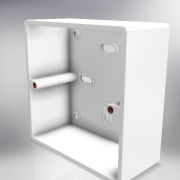
# Autodesk Inventor part: EJB1
Saved by Autodesk Inventor 2020 (Build 240168000, 168)
## iProperties
Created: 2021-02-04
Part Number: EJB1
Material: ABS Plastic
Document SubType Name: Modeling
Designer: Sikesh Bhivah
Mass: 50.6029 g
Surface Area: 410.777 cm^2
Volume: 47.7386 cm^3
Density: 1.06 g/cm^3
Appearance: White
Categories: <MemberInstance><Categories><Category DisplayName="" Mnemonic="IDF" InternalName="690189fb-5335-48bc-ba8f-fa4ddabb13bb"><Category DisplayName="" Mnemonic="COMPONENTS" InternalName="eab5d76b-1861-4102-82a0-277eae840d4a"><Category DisplayName="" Mnemonic="ELECTRICAL" InternalName="e935d458-c05c-4f25-8523-65af19dfc39b"/></Category></Category></Categories><FamilyTemplate><FamilyTemplateParameters></FamilyTemplateParameters></FamilyTemplate><CategoryParameterMap><ParamToTemplateMap></ParamToTemplateMap></CategoryParameterMap></MemberInstance>
Author: Sikesh Bhivah
Autodesk Inventor part; units mm, degrees
ref_plane "YZ Plane" through (0, 0, 0) normal (1, 0, 0) x (0, 1, 0)
ref_plane "XZ Plane" through (0, 0, 0) normal (0, 1, 0) x (-1, 0, 0)
ref_plane "XY Plane" through (0, 0, 0) normal (0, 0, 1) x (1, 0, 0)
sketch "Sketch1" plane through (0, 0, 0) normal (0, 0, 1) x (1, 0, 0)
  line L0 (-40, -43) -> (40, -43)
  line L1 (43, -40) -> (43, 40)
  line L2 (40, 43) -> (-40, 43)
  line L3 (-43, 40) -> (-43, -40)
  line L4 (-43, -43) -> (43, 43) construction
  line L5 (43, -43) -> (-43, 43) construction
  arc A0 (-40, 43) -> (-43, 40) centre (-40, 40) ccw
  arc A1 (43, 40) -> (40, 43) centre (40, 40) ccw
  arc A2 (40, -43) -> (43, -40) centre (40, -40) ccw
  arc A3 (-43, -40) -> (-40, -43) centre (-40, -40) ccw
  point P0 (0, 0)
  dimension "d0" = 86
  dimension "d1" = 3
  dimension "d16" = 86
  constraints: 12 end point, 8 point on circle, 8 point on line, 8 tangent, 4 centre point, 3 equal radius, 2 midpoint, 2 parallel, 1 horizontal, 1 perpendicular
  measures "d0" distance of L4.end L5.end
  measures "d1" radius of A0
  measures "d16" distance between parallel lines of L0 L2
extrude "Extrusion1" add sketch "Sketch1" along normal blind 3
sketch "Sketch2" plane through (0, 0, 3) normal (0, 0, 1) x (1, 0, 0)
  arc A0 (-40, 43) -> (-43, 40) centre (-40, 40) ccw projected
  line L0 (-43, 40) -> (-43, -40) projected
  arc A1 (-43, -40) -> (-40, -43) centre (-40, -40) ccw projected
  line L1 (-40, -43) -> (40, -43) projected
  arc A2 (40, -43) -> (43, -40) centre (40, -40) ccw projected
  line L2 (43, -40) -> (43, 40) projected
  arc A3 (43, 40) -> (40, 43) centre (40, 40) ccw projected
  line L3 (40, 43) -> (-40, 43) projected
  line L4 (-40, -40) -> (-40, 40)
  line L5 (-40, 40) -> (40, 40)
  line L6 (40, 40) -> (40, -40)
  line L7 (40, -40) -> (-40, -40)
  arc A4 (-34, -3) -> (-34, 3) centre (-34, 0) ccw
  arc A5 (34, 3) -> (34, -3) centre (34, 0) ccw
  line L8 (-34, 3) -> (-40, 3)
  line L9 (-34, -3) -> (-40, -3)
  line L10 (34, 3) -> (40, 3)
  line L11 (34, -3) -> (40, -3)
  arc A6 (-34, 3) -> (-34, -3) centre (-34, 0) ccw construction
  arc A7 (34, -3) -> (34, 3) centre (34, 0) ccw construction
  point P0 (0, 0)
  point P1 (40, 0)
  dimension "d4" = 3
  dimension "d5" = 6
  dimension "d6" = 6
  constraints: 16 end point, 10 point on circle, 10 point on line, 4 centre point, 2 equal length, 2 horizontal alignment, 2 perpendicular, 1 equal radius, 1 midpoint, 1 tangent, 3 other
  measures "d4" distance between parallel lines of L0 L4
  measures "d5" diameter of A5
  measures "d6" distance of point (40, 0) A5.centre
extrude "Extrusion2" add sketch "Sketch2" along normal blind 35 contours L3 A3 L2 A2 L1 A1 L0 A0 | L4 L8 A4 L9 | L11 A5 L10 L6
sketch "Sketch3" plane through (0, 0, 38) normal (0, 0, 1) x (1, 0, 0)
  arc A0 (-34, -3) -> (-34, 3) centre (-34, 0) ccw projected
  arc A1 (34, 3) -> (34, -3) centre (34, 0) ccw projected
  arc A2 (-34, -3) -> (-34, 3) centre (-34, 0) ccw projected
  point P0 (0, 0)
  constraints: 2 coincident
hole "Hole1" at (-34, 0, 38) at (34, 0, 38) direction (0, 0, -1) diameter 2.459 depth 18 tip angle 118 countersink diameter 4 countersink angle 90 thread size "M3x0.5" class "6H" standard "ISO Metric profile"
chamfer "Chamfer1" distance 0.3 angle 45 28 edges at (0, 43, 38) (-42.1213, 42.1213, 38) (-43, 0, 38) (-42.1213, -42.1213, 38) (0, -43, 38) (42.1213, -42.1213, 38) (43, 0, 38) (42.1213, 42.1213, 38) (0, 40, 38) (-40, 21.5, 38) (-31, 0, 38) (-37, 3, 38) (-37, -3, 38) (-40, -21.5, 38) (0, -40, 38) (40, -21.5, 38) (40, 21.5, 38) (37, 3, 38) (31, 0, 38) (37, -3, 38) (43, 0, 0) (42.1213, 42.1213, 0) (0, 43, 0) (-42.1213, 42.1213, 0) (-43, 0, 0) (-42.1213, -42.1213, 0) (0, -43, 0) (42.1213, -42.1213, 0)
sketch "Sketch4" plane through (0, 0, 0) normal (0, 0, -1) x (-1, 0, 0)
  line L0 (-8, 21) -> (-4, 21) construction
  line L1 (8, 21) -> (8, 29) construction
  line L2 (8, 29) -> (4, 29) construction
  line L3 (-8, 29) -> (-8, 21) construction
  line L4 (-8, 21) -> (8, 29) construction
  line L5 (8, 21) -> (-8, 29) construction
  line L6 (0, 0) -> (0, 25) construction
  arc A0 (-4, 29) -> (-4, 21) centre (-4, 25) ccw
  line L7 (-4, 21) -> (4, 21)
  line L8 (-4, 29) -> (-8, 29) construction
  arc A1 (-4, 21) -> (-4, 29) centre (-4, 25) ccw construction
  arc A2 (4, 21) -> (4, 29) centre (4, 25) ccw
  line L9 (4, 29) -> (-4, 29)
  line L10 (4, 21) -> (8, 21) construction
  line L11 (-42.7, -40) -> (-42.7, 40) projected
  arc A3 (-42.7, -40) -> (-40, -42.7) centre (-40, -40) ccw projected
  line L12 (40, -42.7) -> (-40, -42.7) projected
  arc A4 (40, -42.7) -> (42.7, -40) centre (40, -40) ccw projected
  line L13 (42.7, 40) -> (42.7, -40) projected
  arc A5 (42.7, 40) -> (40, 42.7) centre (40, 40) ccw projected
  line L14 (-40, 42.7) -> (40, 42.7) projected
  arc A6 (-40, 42.7) -> (-42.7, 40) centre (-40, 40) ccw projected
  line L15 (-39.7, 39.7) -> (-39.7, -39.7)
  line L16 (-39.7, -39.7) -> (39.7, -39.7)
  line L17 (39.7, -39.7) -> (39.7, 39.7)
  line L18 (39.7, 39.7) -> (-39.7, 39.7)
  line L19 (0, -39.7) -> (0, -34) construction
  line L20 (-4, -29) -> (4, -29) construction
  line L21 (4, -29) -> (4, -25) construction
  line L22 (4, -13) -> (-4, -13) construction
  line L23 (-4, -13) -> (-4, -17) construction
  line L24 (-4, -29) -> (4, -13) construction
  line L25 (4, -29) -> (-4, -13) construction
  arc A7 (-4, -17) -> (4, -17) centre (0, -17) ccw construction
  line L26 (4, -17) -> (4, -13) construction
  arc A8 (4, -17) -> (-4, -17) centre (0, -17) ccw
  arc A9 (-4, -25) -> (4, -25) centre (0, -25) ccw
  line L27 (-4, -17) -> (-4, -25)
  line L28 (-4, -25) -> (-4, -29) construction
  line L29 (4, -25) -> (4, -17)
  line L30 (0, 0) -> (0, -13) construction
  circle A10 centre (-31.7, 31.7) radius 4
  circle A11 centre (31.7, 31.7) radius 4
  line L31 (-21, -8) -> (-21, -4) construction
  line L32 (-21, 8) -> (-29, 8) construction
  line L33 (-29, 8) -> (-29, 4) construction
  line L34 (-21, -4) -> (-21, 4)
  line L35 (-29, 4) -> (-29, -4)
  line L36 (-29, -8) -> (-21, -8) construction
  line L37 (-29, -4) -> (-29, -8) construction
  line L38 (-21, 8) -> (-29, -8) construction
  arc A12 (-29, -4) -> (-21, -4) centre (-25, -4) ccw
  arc A13 (-21, -4) -> (-29, -4) centre (-25, -4) ccw construction
  line L39 (-21, -8) -> (-29, 8) construction
  line L40 (-21, 4) -> (-21, 8) construction
  arc A14 (-21, 4) -> (-29, 4) centre (-25, 4) ccw
  line L41 (0, 0) -> (-25, 0) construction
  line L42 (0, 0) -> (13, 0) construction
  line L43 (13, -4) -> (17, -4) construction
  arc A15 (17, 4) -> (17, -4) centre (17, 0) ccw
  line L44 (13, 4) -> (13, -4) construction
  arc A16 (17, -4) -> (17, 4) centre (17, 0) ccw construction
  line L45 (17, 4) -> (13, 4) construction
  line L46 (17, -4) -> (25, -4)
  line L47 (25, 4) -> (17, 4)
  line L48 (29, -4) -> (13, 4) construction
  line L49 (29, 4) -> (13, -4) construction
  line L50 (25, -4) -> (29, -4) construction
  line L51 (29, -4) -> (29, 4) construction
  arc A17 (25, -4) -> (25, 4) centre (25, 0) ccw
  line L52 (29, 4) -> (25, 4) construction
  circle A18 centre (-31.7, -31.7) radius 4
  circle A19 centre (31.7, -31.7) radius 4
  point P0 (0, -21)
  point P1 (0, -21)
  point P2 (0, 21)
  point P3 (-21, 0)
  point P4 (21, 0)
  point P5 (21, 0)
  dimension "d20" = 8
  dimension "d24" = 4
  dimension "d25" = 25
  dimension "d30" = 13
  dimension "d36" = 3
  dimension "d37" = 8
  dimension "d44" = 90
  dimension "d56" = 8
  dimension "d57" = 8
  constraints: 98 end point, 28 tangent, 27 point on circle, 20 parallel, 16 centre point, 12 midpoint, 6 perpendicular, 6 symmetric about line, 4 horizontal, 3 equal length, 2 equal radius, 1 coincident, 1 vertical, 1 vertical alignment, 63 other
  measures "d20" distance of A2.centre A0.centre
  measures "d24" radius of A0
  measures "d25" distance of L6.start point (0, 25)
  measures "d30" distance of L6.start L30.end
  measures "d36" distance between parallel lines of L11 L15
  measures "d37" diameter of A10
  measures "d56" distance from line of L18 A10.centre
  measures "d57" distance from line of L15 A10.centre
extrude "Extrusion3" cut sketch "Sketch4" against normal blind 1 contours L18 L17 L16 L15 | A18 | A19
sketch "Sketch5" plane through (0, 0, 3) normal (0, 0, 1) x (1, 0, 0)
  line L0 (4, 21) -> (-4, 21) projected
  arc A0 (-4, 29) -> (-4, 21) centre (-4, 25) ccw projected
  line L1 (-4, 29) -> (4, 29) projected
  arc A1 (4, 21) -> (4, 29) centre (4, 25) ccw projected
  circle A2 centre (-31.7, 31.7) radius 4 projected
  arc A3 (4, -17) -> (-4, -17) centre (0, -17) ccw projected
  line L2 (4, -17) -> (4, -25) projected
  arc A4 (-4, -25) -> (4, -25) centre (0, -25) ccw projected
  line L3 (-4, -25) -> (-4, -17) projected
  circle A5 centre (31.7, 31.7) radius 4 projected
  circle A6 centre (31.9662, -31.9095) radius 4 projected
  circle A7 centre (-31.9662, -31.9095) radius 4 projected
  line L4 (-40, 40) -> (-40, 3) projected
  line L5 (-40, 3) -> (-34, 3) projected
  arc A8 (-34, -3) -> (-34, 3) centre (-34, 0) ccw projected
  line L6 (-34, -3) -> (-40, -3) projected
  line L7 (-40, -3) -> (-40, -40) projected
  line L8 (-40, -40) -> (40, -40) projected
  line L9 (40, -40) -> (40, -3) projected
  line L10 (40, -3) -> (34, -3) projected
  arc A9 (34, 3) -> (34, -3) centre (34, 0) ccw projected
  line L11 (34, 3) -> (40, 3) projected
  line L12 (40, 3) -> (40, 40) projected
  line L13 (40, 40) -> (-40, 40) projected
  arc A10 (29, 4) -> (21, 4) centre (25, 4) ccw projected
  line L14 (29, 4) -> (29, -4) projected
  arc A11 (21, -4) -> (29, -4) centre (25, -4) ccw projected
  line L15 (21, -4) -> (21, 4) projected
  arc A12 (-25, 4) -> (-25, -4) centre (-25, 0) ccw projected
  line L16 (-25, 4) -> (-17, 4) projected
  arc A13 (-17, -4) -> (-17, 4) centre (-17, 0) ccw projected
  line L17 (-17, -4) -> (-25, -4) projected
  point P0 (0, 0)
extrude "Extrusion4" cut sketch "Sketch5" against normal blind 1
sketch "Sketch6" plane through (-31.7, 31.7, 3) normal (0, 0, 1) x (1, 0, 0)
  circle A0 centre (0, 0) radius 4 projected
  arc A1 (35.7, -10.7) -> (35.7, -2.7) centre (35.7, -6.7) ccw projected
  line L0 (35.7, -2.7) -> (27.7, -2.7) projected
  arc A2 (27.7, -2.7) -> (27.7, -10.7) centre (27.7, -6.7) ccw projected
  line L1 (27.7, -10.7) -> (35.7, -10.7) projected
  circle A3 centre (63.4, 0) radius 4 projected
  arc A4 (60.7, -27.7) -> (52.7, -27.7) centre (56.7, -27.7) ccw projected
  line L2 (52.7, -27.7) -> (52.7, -35.7) projected
  arc A5 (52.7, -35.7) -> (60.7, -35.7) centre (56.7, -35.7) ccw projected
  line L3 (60.7, -35.7) -> (60.7, -27.7) projected
  arc A6 (27.7, -56.7) -> (35.7, -56.7) centre (31.7, -56.7) ccw projected
  line L4 (35.7, -56.7) -> (35.7, -48.7) projected
  arc A7 (35.7, -48.7) -> (27.7, -48.7) centre (31.7, -48.7) ccw projected
  line L5 (27.7, -48.7) -> (27.7, -56.7) projected
  arc A8 (6.7, -27.7) -> (6.7, -35.7) centre (6.7, -31.7) ccw projected
  line L6 (6.7, -35.7) -> (14.7, -35.7) projected
  arc A9 (14.7, -35.7) -> (14.7, -27.7) centre (14.7, -31.7) ccw projected
  line L7 (14.7, -27.7) -> (6.7, -27.7) projected
  circle A10 centre (-0.2662, -63.6095) radius 4 projected
  circle A11 centre (63.6662, -63.6095) radius 4 projected
  circle A12 centre (0, 0) radius 2.5
  line L8 (27.7, -4.2) -> (35.7, -4.2)
  arc A13 (35.7, -9.2) -> (35.7, -4.2) centre (35.7, -6.7) ccw
  line L9 (35.7, -9.2) -> (27.7, -9.2)
  arc A14 (27.7, -4.2) -> (27.7, -9.2) centre (27.7, -6.7) ccw
  line L10 (34.2, -48.7) -> (34.2, -56.7)
  arc A15 (29.2, -56.7) -> (34.2, -56.7) centre (31.7, -56.7) ccw
  line L11 (29.2, -56.7) -> (29.2, -48.7)
  arc A16 (34.2, -48.7) -> (29.2, -48.7) centre (31.7, -48.7) ccw
  arc A17 (14.7, -34.2) -> (14.7, -29.2) centre (14.7, -31.7) ccw
  line L12 (14.7, -34.2) -> (6.7, -34.2)
  arc A18 (6.7, -29.2) -> (6.7, -34.2) centre (6.7, -31.7) ccw
  line L13 (6.7, -29.2) -> (14.7, -29.2)
  arc A19 (54.2, -35.7) -> (59.2, -35.7) centre (56.7, -35.7) ccw
  line L14 (54.2, -35.7) -> (54.2, -27.7)
  arc A20 (59.2, -27.7) -> (54.2, -27.7) centre (56.7, -27.7) ccw
  line L15 (59.2, -27.7) -> (59.2, -35.7)
  circle A21 centre (63.4, 0) radius 2.5
  circle A22 centre (-0.2662, -63.6095) radius 2.5
  circle A23 centre (63.6662, -63.6095) radius 2.5
  point P0 (31.7, -31.7)
  dimension "d46" = 1.5
  dimension "d47" = 1.5
  dimension "d48" = 1.5
  dimension "d49" = 1.5
  dimension "d50" = 1.5
  dimension "d51" = 1.5
  dimension "d52" = 1.5
  dimension "d53" = 1.5
  constraints: 16 end point, 16 point on circle, 12 centre point, 12 other
  measures "d46" radial gap between concentric circles of A0 A12
  measures "d47" distance between parallel lines of L0 L8
  measures "d48" distance between parallel lines of L4 L10
  measures "d49" radial gap between concentric circles of A9 A17
  measures "d50" radial gap between concentric circles of A5 A19
  measures "d51" radial gap between concentric circles of A3 A21
  measures "d52" radial gap between concentric circles of A10 A22
  measures "d53" radial gap between concentric circles of A11 A23
extrude "Extrusion5" cut sketch "Sketch6" against normal through all contours A12 | L8 A13 L9 A14 | L10 A15 L11 A16 | L12 A18 L13 A17 | L14 A20 L15 A19 | A21 | A22 | A23
equation "\"d0\" = Width"
equation "\"d2\" = d1"
equation "\"d6\" = d5"
equation "\"d7\" = Depth"
equation "\"d37\" = 2 * d24"
equation "\"d57\" = d37"
equation "\"d47\" = d46"
equation "\"d48\" = d50"
equation "\"d49\" = d51"
equation "\"d50\" = d49"
equation "\"d51\" = d47"
equation "\"d52\" = d53"
equation "\"d53\" = d48"
equation "\"Depth\" = 35"
equation "\"Width\" = 86"
body "Solid1"
